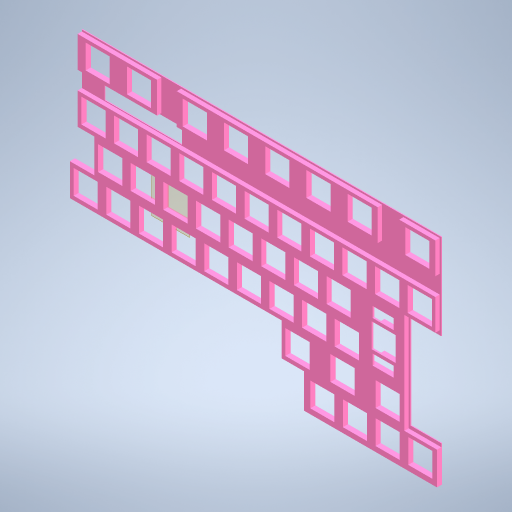
# Autodesk Inventor part: Upper Right Plate
Saved by Autodesk Inventor 2024 (Build 280153000, 153)
## iProperties
Created: 2024-06-29
Part Number: Upper Right Plate
Material: PET Plastic
Document SubType Name: Modeling
Designer: adam
Density: 1.541 g/cm^3
Appearance: Pink
Author: adam
Autodesk Inventor part; units mm, degrees
(part 1 of 2)
ref_plane "YZ Plane" through (0, 0, 0) normal (1, 0, 0) x (0, 1, 0)
ref_plane "XZ Plane" through (0, 0, 0) normal (0, 1, 0) x (-1, 0, 0)
ref_plane "XY Plane" through (0, 0, 0) normal (0, 0, 1) x (1, 0, 0)
sketch "Sketch1" plane through (0, 0, 0) normal (0, 0, 1) x (1, 0, 0)
  line L0 (43.325, -43.95) -> (49.375, -43.95) construction
  line L1 (49.375, -43.95) -> (49.375, -61) construction
  line L2 (49.375, -61) -> (43.325, -61) construction
  line L3 (43.325, -61) -> (43.325, -43.95) construction
  line L4 (117.95, -19.8) -> (117.95, -13.75) construction
  line L5 (117.95, -13.75) -> (135, -13.75) construction
  line L6 (135, -13.75) -> (135, -19.8) construction
  line L7 (135, -19.8) -> (117.95, -19.8) construction
  line L8 (26.325, -43.95) -> (32.375, -43.95) construction
  line L9 (32.375, -43.95) -> (32.375, -61) construction
  line L10 (32.375, -61) -> (26.325, -61) construction
  line L11 (26.325, -61) -> (26.325, -43.95) construction
  line L12 (-152.525, 13.425) -> (-146.475, 13.425) construction
  line L13 (-146.475, 13.425) -> (-146.475, -3.625) construction
  line L14 (-146.475, -3.625) -> (-152.525, -3.625) construction
  line L15 (-152.525, -3.625) -> (-152.525, 13.425) construction
  line L16 (-90.675, -43.95) -> (-84.625, -43.95) construction
  line L17 (-84.625, -43.95) -> (-84.625, -61) construction
  line L18 (-84.625, -61) -> (-90.675, -61) construction
  line L19 (-90.675, -61) -> (-90.675, -43.95) construction
  line L20 (39.375, -43.95) -> (39.375, -61) construction
  line L21 (39.375, -61) -> (33.325, -61) construction
  line L22 (33.325, -61) -> (33.325, -43.95) construction
  line L23 (33.325, -43.95) -> (39.375, -43.95) construction
  line L24 (117.95, 4.2) -> (117.95, 10.25) construction
  line L25 (117.95, 10.25) -> (135, 10.25) construction
  line L26 (135, 10.25) -> (135, 4.2) construction
  line L27 (135, 4.2) -> (117.95, 4.2) construction
  line L28 (-67.625, -43.95) -> (-67.625, -61) construction
  line L29 (-67.625, -61) -> (-73.675, -61) construction
  line L30 (-73.675, -61) -> (-73.675, -43.95) construction
  line L31 (-73.675, -43.95) -> (-67.625, -43.95) construction
  line L32 (-128.525, 13.425) -> (-122.475, 13.425) construction
  line L33 (-122.475, 13.425) -> (-122.475, -3.625) construction
  line L34 (-122.475, -3.625) -> (-128.525, -3.625) construction
  line L35 (-128.525, -3.625) -> (-128.525, 13.425) construction
  line L36 (-74.625, -43.95) -> (-74.625, -61) construction
  line L37 (-74.625, -61) -> (-80.675, -61) construction
  line L38 (-80.675, -61) -> (-80.675, -43.95) construction
  line L39 (-80.675, -43.95) -> (-74.625, -43.95) construction
  line L40 (-157.5, -62.5) -> (157.5, -62.5) construction
  line L41 (157.5, -62.5) -> (157.5, -41.5) construction
  line L42 (157.5, -41.5) -> (139.5, -41.5) construction
  line L43 (139.5, -41.5) -> (139.5, 12.5) construction
  line L44 (139.5, 12.5) -> (157.5, 12.5) construction
  line L45 (157.5, 12.5) -> (157.5, 62.5) construction
  line L46 (157.5, 62.5) -> (-157.5, 62.5) construction
  line L47 (-157.5, 62.5) -> (-157.5, -62.5) construction
  line L48 (-38.5, 42.5) -> (6.5, 42.5) construction
  line L49 (6.5, 42.5) -> (6.5, 33.5) construction
  line L50 (6.5, 33.5) -> (-38.5, 33.5) construction
  line L51 (-38.5, 33.5) -> (-38.5, 42.5) construction
  line L52 (154.775, -45.45) -> (154.775, -59.5) construction
  line L53 (154.775, -59.5) -> (140.725, -59.5) construction
  line L54 (140.725, -59.5) -> (140.725, -45.45) construction
  line L55 (140.725, -45.45) -> (154.775, -45.45) construction
  line L56 (135.775, -45.45) -> (135.775, -59.5) construction
  line L57 (135.775, -59.5) -> (121.725, -59.5) construction
  line L58 (121.725, -59.5) -> (121.725, -45.45) construction
  line L59 (121.725, -45.45) -> (135.775, -45.45) construction
  line L60 (116.775, -45.45) -> (116.775, -59.5) construction
  line L61 (116.775, -59.5) -> (102.725, -59.5) construction
  line L62 (102.725, -59.5) -> (102.725, -45.45) construction
  line L63 (102.725, -45.45) -> (116.775, -45.45) construction
  line L64 (97.775, -45.45) -> (97.775, -59.5) construction
  line L65 (97.775, -59.5) -> (83.725, -59.5) construction
  line L66 (83.725, -59.5) -> (83.725, -45.45) construction
  line L67 (83.725, -45.45) -> (97.775, -45.45) construction
  line L68 (75.775, -45.45) -> (75.775, -59.5) construction
  line L69 (75.775, -59.5) -> (61.725, -59.5) construction
  line L70 (61.725, -59.5) -> (61.725, -45.45) construction
  line L71 (61.725, -45.45) -> (75.775, -45.45) construction
  line L72 (-13.625, -45.45) -> (-13.625, -59.5) construction
  line L73 (-13.625, -59.5) -> (-27.675, -59.5) construction
  line L74 (-27.675, -59.5) -> (-27.675, -45.45) construction
  line L75 (-27.675, -45.45) -> (-13.625, -45.45) construction
  line L76 (-102.975, -45.45) -> (-102.975, -59.5) construction
  line L77 (-102.975, -59.5) -> (-117.025, -59.5) construction
  line L78 (-117.025, -59.5) -> (-117.025, -45.45) construction
  line L79 (-117.025, -45.45) -> (-102.975, -45.45) construction
  line L80 (-141.525, -45.45) -> (-127.475, -45.45) construction
  line L81 (-127.475, -45.45) -> (-127.475, -59.5) construction
  line L82 (-127.475, -59.5) -> (-141.525, -59.5) construction
  line L83 (-141.525, -59.5) -> (-141.525, -45.45) construction
  line L84 (121.725, -26.275) -> (135.775, -26.275) construction
  line L85 (135.775, -26.275) -> (135.775, -40.325) construction
  line L86 (135.775, -40.325) -> (121.725, -40.325) construction
  line L87 (121.725, -40.325) -> (121.725, -26.275) construction
  line L88 (95.475, -26.275) -> (109.525, -26.275) construction
  line L89 (109.525, -26.275) -> (109.525, -40.325) construction
  line L90 (109.525, -40.325) -> (95.475, -40.325) construction
  line L91 (95.475, -40.325) -> (95.475, -26.275) construction
  line L92 (69.225, -26.275) -> (83.275, -26.275) construction
  line L93 (83.275, -26.275) -> (83.275, -40.325) construction
  line L94 (83.275, -40.325) -> (69.225, -40.325) construction
  line L95 (69.225, -40.325) -> (69.225, -26.275) construction
  line L96 (50.225, -26.275) -> (64.275, -26.275) construction
  line L97 (64.275, -26.275) -> (64.275, -40.325) construction
  line L98 (64.275, -40.325) -> (50.225, -40.325) construction
  line L99 (50.225, -40.325) -> (50.225, -26.275) construction
  line L100 (31.225, -26.275) -> (45.275, -26.275) construction
  line L101 (45.275, -26.275) -> (45.275, -40.325) construction
  line L102 (45.275, -40.325) -> (31.225, -40.325) construction
  line L103 (31.225, -40.325) -> (31.225, -26.275) construction
  line L104 (12.225, -26.275) -> (26.275, -26.275) construction
  line L105 (26.275, -26.275) -> (26.275, -40.325) construction
  line L106 (26.275, -40.325) -> (12.225, -40.325) construction
  line L107 (12.225, -40.325) -> (12.225, -26.275) construction
  line L108 (-6.775, -26.275) -> (7.275, -26.275) construction
  line L109 (7.275, -26.275) -> (7.275, -40.325) construction
  line L110 (7.275, -40.325) -> (-6.775, -40.325) construction
  line L111 (-6.775, -40.325) -> (-6.775, -26.275) construction
  line L112 (-25.775, -26.275) -> (-11.725, -26.275) construction
  line L113 (-11.725, -26.275) -> (-11.725, -40.325) construction
  line L114 (-11.725, -40.325) -> (-25.775, -40.325) construction
  line L115 (-25.775, -40.325) -> (-25.775, -26.275) construction
  line L116 (-44.775, -26.275) -> (-30.725, -26.275) construction
  line L117 (-30.725, -26.275) -> (-30.725, -40.325) construction
  line L118 (-30.725, -40.325) -> (-44.775, -40.325) construction
  line L119 (-44.775, -40.325) -> (-44.775, -26.275) construction
  line L120 (-63.775, -26.275) -> (-49.725, -26.275) construction
  line L121 (-49.725, -26.275) -> (-49.725, -40.325) construction
  line L122 (-49.725, -40.325) -> (-63.775, -40.325) construction
  line L123 (-63.775, -40.325) -> (-63.775, -26.275) construction
  line L124 (-82.775, -26.275) -> (-68.725, -26.275) construction
  line L125 (-68.725, -26.275) -> (-68.725, -40.325) construction
  line L126 (-68.725, -40.325) -> (-82.775, -40.325) construction
  line L127 (-82.775, -40.325) -> (-82.775, -26.275) construction
  line L128 (-101.775, -26.275) -> (-87.725, -26.275) construction
  line L129 (-87.725, -26.275) -> (-87.725, -40.325) construction
  line L130 (-87.725, -40.325) -> (-101.775, -40.325) construction
  line L131 (-101.775, -40.325) -> (-101.775, -26.275) construction
  line L132 (-120.775, -26.275) -> (-106.725, -26.275) construction
  line L133 (-106.725, -26.275) -> (-106.725, -40.325) construction
  line L134 (-106.725, -40.325) -> (-120.775, -40.325) construction
  line L135 (-120.775, -40.325) -> (-120.775, -26.275) construction
  line L136 (-146.775, -26.275) -> (-132.725, -26.275) construction
  line L137 (-132.725, -26.275) -> (-132.725, -40.325) construction
  line L138 (-132.725, -40.325) -> (-146.775, -40.325) construction
  line L139 (-146.775, -40.325) -> (-146.775, -26.275) construction
  line L140 (97.975, -7.175) -> (112.025, -7.175) construction
  line L141 (112.025, -7.175) -> (112.025, -21.225) construction
  line L142 (112.025, -21.225) -> (97.975, -21.225) construction
  line L143 (97.975, -21.225) -> (97.975, -7.175) construction
  line L144 (78.975, -7.175) -> (93.025, -7.175) construction
  line L145 (93.025, -7.175) -> (93.025, -21.225) construction
  line L146 (93.025, -21.225) -> (78.975, -21.225) construction
  line L147 (78.975, -21.225) -> (78.975, -7.175) construction
  line L148 (59.975, -7.175) -> (74.025, -7.175) construction
  line L149 (74.025, -7.175) -> (74.025, -21.225) construction
  line L150 (74.025, -21.225) -> (59.975, -21.225) construction
  line L151 (59.975, -21.225) -> (59.975, -7.175) construction
  line L152 (40.975, -7.175) -> (55.025, -7.175) construction
  line L153 (55.025, -7.175) -> (55.025, -21.225) construction
  line L154 (55.025, -21.225) -> (40.975, -21.225) construction
  line L155 (40.975, -21.225) -> (40.975, -7.175) construction
  line L156 (21.975, -7.175) -> (36.025, -7.175) construction
  line L157 (36.025, -7.175) -> (36.025, -21.225) construction
  line L158 (36.025, -21.225) -> (21.975, -21.225) construction
  line L159 (21.975, -21.225) -> (21.975, -7.175) construction
  line L160 (2.975, -7.175) -> (17.025, -7.175) construction
  line L161 (17.025, -7.175) -> (17.025, -21.225) construction
  line L162 (17.025, -21.225) -> (2.975, -21.225) construction
  line L163 (2.975, -21.225) -> (2.975, -7.175) construction
  line L164 (-16.025, -7.175) -> (-1.975, -7.175) construction
  line L165 (-1.975, -7.175) -> (-1.975, -21.225) construction
  line L166 (-1.975, -21.225) -> (-16.025, -21.225) construction
  line L167 (-16.025, -21.225) -> (-16.025, -7.175) construction
  line L168 (-35.025, -7.175) -> (-20.975, -7.175) construction
  line L169 (-20.975, -7.175) -> (-20.975, -21.225) construction
  line L170 (-20.975, -21.225) -> (-35.025, -21.225) construction
  line L171 (-35.025, -21.225) -> (-35.025, -7.175) construction
  line L172 (-54.025, -7.175) -> (-39.975, -7.175) construction
  line L173 (-39.975, -7.175) -> (-39.975, -21.225) construction
  line L174 (-39.975, -21.225) -> (-54.025, -21.225) construction
  line L175 (-54.025, -21.225) -> (-54.025, -7.175) construction
  line L176 (-73.025, -7.175) -> (-58.975, -7.175) construction
  line L177 (-58.975, -7.175) -> (-58.975, -21.225) construction
  line L178 (-58.975, -21.225) -> (-73.025, -21.225) construction
  line L179 (-73.025, -21.225) -> (-73.025, -7.175) construction
  line L180 (-92.025, -7.175) -> (-77.975, -7.175) construction
  line L181 (-77.975, -7.175) -> (-77.975, -21.225) construction
  line L182 (-77.975, -21.225) -> (-92.025, -21.225) construction
  line L183 (-92.025, -21.225) -> (-92.025, -7.175) construction
  line L184 (-111.025, -7.175) -> (-96.975, -7.175) construction
  line L185 (-96.975, -7.175) -> (-96.975, -21.225) construction
  line L186 (-96.975, -21.225) -> (-111.025, -21.225) construction
  line L187 (-111.025, -21.225) -> (-111.025, -7.175) construction
  line L188 (-130.025, -7.175) -> (-115.975, -7.175) construction
  line L189 (-115.975, -7.175) -> (-115.975, -21.225) construction
  line L190 (-115.975, -21.225) -> (-130.025, -21.225) construction
  line L191 (-130.025, -21.225) -> (-130.025, -7.175) construction
  line L192 (-151.525, -7.175) -> (-137.475, -7.175) construction
  line L193 (-137.475, -7.175) -> (-137.475, -21.225) construction
  line L194 (-137.475, -21.225) -> (-151.525, -21.225) construction
  line L195 (-151.525, -21.225) -> (-151.525, -7.175) construction
  line L196 (119.45, 2.25) -> (133.5, 2.25) construction
  line L197 (133.5, 2.25) -> (133.5, -11.8) construction
  line L198 (133.5, -11.8) -> (119.45, -11.8) construction
  line L199 (119.45, -11.8) -> (119.45, 2.25) construction
  line L200 (107.275, 11.925) -> (107.275, -2.125) construction
  line L201 (107.275, -2.125) -> (93.225, -2.125) construction
  line L202 (93.225, -2.125) -> (93.225, 11.925) construction
  line L203 (93.225, 11.925) -> (107.275, 11.925) construction
  line L204 (88.275, 11.925) -> (88.275, -2.125) construction
  line L205 (88.275, -2.125) -> (74.225, -2.125) construction
  line L206 (74.225, -2.125) -> (74.225, 11.925) construction
  line L207 (74.225, 11.925) -> (88.275, 11.925) construction
  line L208 (69.275, 11.925) -> (69.275, -2.125) construction
  line L209 (69.275, -2.125) -> (55.225, -2.125) construction
  line L210 (55.225, -2.125) -> (55.225, 11.925) construction
  line L211 (55.225, 11.925) -> (69.275, 11.925) construction
  line L212 (50.275, 11.925) -> (50.275, -2.125) construction
  line L213 (50.275, -2.125) -> (36.225, -2.125) construction
  line L214 (36.225, -2.125) -> (36.225, 11.925) construction
  line L215 (36.225, 11.925) -> (50.275, 11.925) construction
  line L216 (31.275, 11.925) -> (31.275, -2.125) construction
  line L217 (31.275, -2.125) -> (17.225, -2.125) construction
  line L218 (17.225, -2.125) -> (17.225, 11.925) construction
  line L219 (17.225, 11.925) -> (31.275, 11.925) construction
  line L220 (12.275, 11.925) -> (12.275, -2.125) construction
  line L221 (12.275, -2.125) -> (-1.775, -2.125) construction
  line L222 (-1.775, -2.125) -> (-1.775, 11.925) construction
  line L223 (-1.775, 11.925) -> (12.275, 11.925) construction
  line L224 (-6.725, 11.925) -> (-6.725, -2.125) construction
  line L225 (-6.725, -2.125) -> (-20.775, -2.125) construction
  line L226 (-20.775, -2.125) -> (-20.775, 11.925) construction
  line L227 (-20.775, 11.925) -> (-6.725, 11.925) construction
  line L228 (-25.725, 11.925) -> (-25.725, -2.125) construction
  line L229 (-25.725, -2.125) -> (-39.775, -2.125) construction
  line L230 (-39.775, -2.125) -> (-39.775, 11.925) construction
  line L231 (-39.775, 11.925) -> (-25.725, 11.925) construction
  line L232 (-44.725, 11.925) -> (-44.725, -2.125) construction
  line L233 (-44.725, -2.125) -> (-58.775, -2.125) construction
  line L234 (-58.775, -2.125) -> (-58.775, 11.925) construction
  line L235 (-58.775, 11.925) -> (-44.725, 11.925) construction
  line L236 (-63.725, 11.925) -> (-63.725, -2.125) construction
  line L237 (-63.725, -2.125) -> (-77.775, -2.125) construction
  line L238 (-77.775, -2.125) -> (-77.775, 11.925) construction
  line L239 (-77.775, 11.925) -> (-63.725, 11.925) construction
  line L240 (-82.725, 11.925) -> (-82.725, -2.125) construction
  line L241 (-82.725, -2.125) -> (-96.775, -2.125) construction
  line L242 (-96.775, -2.125) -> (-96.775, 11.925) construction
  line L243 (-96.775, 11.925) -> (-82.725, 11.925) construction
  line L244 (-101.725, 11.925) -> (-101.725, -2.125) construction
  line L245 (-101.725, -2.125) -> (-115.775, -2.125) construction
  line L246 (-115.775, -2.125) -> (-115.775, 11.925) construction
  line L247 (-115.775, 11.925) -> (-101.725, 11.925) construction
  line L248 (-144.525, 11.925) -> (-130.475, 11.925) construction
  line L249 (-130.475, 11.925) -> (-130.475, -2.125) construction
  line L250 (-130.475, -2.125) -> (-144.525, -2.125) construction
  line L251 (-144.525, -2.125) -> (-144.525, 11.925) construction
  line L252 (154.525, 16.975) -> (140.475, 16.975) construction
  line L253 (140.475, 16.975) -> (140.475, 31.025) construction
  line L254 (140.475, 31.025) -> (154.525, 31.025) construction
  line L255 (154.525, 31.025) -> (154.525, 16.975) construction
  line L256 (135.525, 16.975) -> (121.475, 16.975) construction
  line L257 (121.475, 16.975) -> (121.475, 31.025) construction
  line L258 (121.475, 31.025) -> (135.525, 31.025) construction
  line L259 (135.525, 31.025) -> (135.525, 16.975) construction
  line L260 (116.525, 16.975) -> (102.475, 16.975) construction
  line L261 (102.475, 16.975) -> (102.475, 31.025) construction
  line L262 (102.475, 31.025) -> (116.525, 31.025) construction
  line L263 (116.525, 31.025) -> (116.525, 16.975) construction
  line L264 (97.525, 16.975) -> (83.475, 16.975) construction
  line L265 (83.475, 16.975) -> (83.475, 31.025) construction
  line L266 (83.475, 31.025) -> (97.525, 31.025) construction
  line L267 (97.525, 31.025) -> (97.525, 16.975) construction
  line L268 (78.525, 16.975) -> (64.475, 16.975) construction
  line L269 (64.475, 16.975) -> (64.475, 31.025) construction
  line L270 (64.475, 31.025) -> (78.525, 31.025) construction
  line L271 (78.525, 31.025) -> (78.525, 16.975) construction
  line L272 (59.525, 16.975) -> (45.475, 16.975) construction
  line L273 (45.475, 16.975) -> (45.475, 31.025) construction
  line L274 (45.475, 31.025) -> (59.525, 31.025) construction
  line L275 (59.525, 31.025) -> (59.525, 16.975) construction
  line L276 (40.525, 16.975) -> (26.475, 16.975) construction
  line L277 (26.475, 16.975) -> (26.475, 31.025) construction
  line L278 (26.475, 31.025) -> (40.525, 31.025) construction
  line L279 (40.525, 31.025) -> (40.525, 16.975) construction
  line L280 (21.525, 16.975) -> (7.475, 16.975) construction
  line L281 (7.475, 16.975) -> (7.475, 31.025) construction
  line L282 (7.475, 31.025) -> (21.525, 31.025) construction
  line L283 (21.525, 31.025) -> (21.525, 16.975) construction
  line L284 (2.525, 16.975) -> (-11.525, 16.975) construction
  line L285 (-11.525, 16.975) -> (-11.525, 31.025) construction
  line L286 (-11.525, 31.025) -> (2.525, 31.025) construction
  line L287 (2.525, 31.025) -> (2.525, 16.975) construction
  line L288 (-16.475, 16.975) -> (-30.525, 16.975) construction
  line L289 (-30.525, 16.975) -> (-30.525, 31.025) construction
  line L290 (-30.525, 31.025) -> (-16.475, 31.025) construction
  line L291 (-16.475, 31.025) -> (-16.475, 16.975) construction
  line L292 (-35.475, 16.975) -> (-49.525, 16.975) construction
  line L293 (-49.525, 16.975) -> (-49.525, 31.025) construction
  line L294 (-49.525, 31.025) -> (-35.475, 31.025) construction
  line L295 (-35.475, 31.025) -> (-35.475, 16.975) construction
  line L296 (-54.475, 16.975) -> (-68.525, 16.975) construction
  line L297 (-68.525, 16.975) -> (-68.525, 31.025) construction
  line L298 (-68.525, 31.025) -> (-54.475, 31.025) construction
  line L299 (-54.475, 31.025) -> (-54.475, 16.975) construction
  line L300 (-73.475, 16.975) -> (-87.525, 16.975) construction
  line L301 (-87.525, 16.975) -> (-87.525, 31.025) construction
  line L302 (-87.525, 31.025) -> (-73.475, 31.025) construction
  line L303 (-73.475, 31.025) -> (-73.475, 16.975) construction
  line L304 (-92.475, 16.975) -> (-106.525, 16.975) construction
  line L305 (-106.525, 16.975) -> (-106.525, 31.025) construction
  line L306 (-106.525, 31.025) -> (-92.475, 31.025) construction
  line L307 (-92.475, 31.025) -> (-92.475, 16.975) construction
  line L308 (-111.475, 16.975) -> (-125.525, 16.975) construction
  line L309 (-125.525, 16.975) -> (-125.525, 31.025) construction
  line L310 (-125.525, 31.025) -> (-111.475, 31.025) construction
  line L311 (-111.475, 31.025) -> (-111.475, 16.975) construction
  line L312 (-149.525, 31.025) -> (-135.475, 31.025) construction
  line L313 (-135.475, 31.025) -> (-135.475, 16.975) construction
  line L314 (-135.475, 16.975) -> (-149.525, 16.975) construction
  line L315 (-149.525, 16.975) -> (-149.525, 31.025) construction
  line L316 (138.975, 59.525) -> (153.025, 59.525) construction
  line L317 (153.025, 59.525) -> (153.025, 45.475) construction
  line L318 (153.025, 45.475) -> (138.975, 45.475) construction
  line L319 (138.975, 45.475) -> (138.975, 59.525) construction
  line L320 (105.475, 59.525) -> (119.525, 59.525) construction
  line L321 (119.525, 59.525) -> (119.525, 45.475) construction
  line L322 (119.525, 45.475) -> (105.475, 45.475) construction
  line L323 (105.475, 45.475) -> (105.475, 59.525) construction
  line L324 (81.475, 59.525) -> (95.525, 59.525) construction
  line L325 (95.525, 59.525) -> (95.525, 45.475) construction
  line L326 (95.525, 45.475) -> (81.475, 45.475) construction
  line L327 (81.475, 45.475) -> (81.475, 59.525) construction
  line L328 (57.475, 59.525) -> (71.525, 59.525) construction
  line L329 (71.525, 59.525) -> (71.525, 45.475) construction
  line L330 (71.525, 45.475) -> (57.475, 45.475) construction
  line L331 (57.475, 45.475) -> (57.475, 59.525) construction
  line L332 (33.475, 59.525) -> (47.525, 59.525) construction
  line L333 (47.525, 59.525) -> (47.525, 45.475) construction
  line L334 (47.525, 45.475) -> (33.475, 45.475) construction
  line L335 (33.475, 45.475) -> (33.475, 59.525) construction
  line L336 (9.475, 59.525) -> (23.525, 59.525) construction
  line L337 (23.525, 59.525) -> (23.525, 45.475) construction
  line L338 (23.525, 45.475) -> (9.475, 45.475) construction
  line L339 (9.475, 45.475) -> (9.475, 59.525) construction
  line L340 (-23.025, 59.525) -> (-8.975, 59.525) construction
  line L341 (-8.975, 59.525) -> (-8.975, 45.475) construction
  line L342 (-8.975, 45.475) -> (-23.025, 45.475) construction
  line L343 (-23.025, 45.475) -> (-23.025, 59.525) construction
  line L344 (-47.025, 59.525) -> (-32.975, 59.525) construction
  line L345 (-32.975, 59.525) -> (-32.975, 45.475) construction
  line L346 (-32.975, 45.475) -> (-47.025, 45.475) construction
  line L347 (-47.025, 45.475) -> (-47.025, 59.525) construction
  line L348 (-71.025, 59.525) -> (-56.975, 59.525) construction
  line L349 (-56.975, 59.525) -> (-56.975, 45.475) construction
  line L350 (-56.975, 45.475) -> (-71.025, 45.475) construction
  line L351 (-71.025, 45.475) -> (-71.025, 59.525) construction
  line L352 (-95.025, 59.525) -> (-80.975, 59.525) construction
  line L353 (-80.975, 59.525) -> (-80.975, 45.475) construction
  line L354 (-80.975, 45.475) -> (-95.025, 45.475) construction
  line L355 (-95.025, 45.475) -> (-95.025, 59.525) construction
  line L356 (-119.025, 59.525) -> (-104.975, 59.525) construction
  line L357 (-104.975, 59.525) -> (-104.975, 45.475) construction
  line L358 (-104.975, 45.475) -> (-119.025, 45.475) construction
  line L359 (-119.025, 45.475) -> (-119.025, 59.525) construction
  line L360 (-152.025, 59.525) -> (-137.975, 59.525) construction
  line L361 (-137.975, 59.525) -> (-137.975, 45.475) construction
  line L362 (-137.975, 45.475) -> (-152.025, 45.475) construction
  line L363 (-152.025, 45.475) -> (-152.025, 59.525) construction
  line L364 (79.5, -62.5) -> (79.5, -43.1375) construction
  line L365 (79.5, -43.1375) -> (66.5, -43.1375) construction
  line L366 (66.5, -43.1375) -> (66.5, -24) construction
  line L367 (66.5, -24) -> (-104, -24) construction
  line L368 (-104, -24) -> (-104, -43.1375) construction
  line L369 (-104, -43.1375) -> (-122, -43.1375) construction
  line L370 (-122, -43.1375) -> (-122, -62.5) construction
  line L371 (-122, -62.5) -> (79.5, -62.5) construction
  line L372 (43.325, -58.35) -> (43.325, -45.95) construction
  line L373 (43.325, -45.95) -> (49.375, -45.95) construction
  line L374 (49.375, -45.95) -> (49.375, -58.35) construction
  line L375 (49.375, -58.35) -> (43.325, -58.35) construction
  line L376 (-90.675, -58.35) -> (-90.675, -45.95) construction
  line L377 (-90.675, -45.95) -> (-84.625, -45.95) construction
  line L378 (-84.625, -45.95) -> (-84.625, -58.35) construction
  line L379 (-84.625, -58.35) -> (-90.675, -58.35) construction
  line L380 (61.725, -45.45) -> (75.775, -45.45) construction
  line L381 (75.775, -45.45) -> (75.775, -59.5) construction
  line L382 (75.775, -59.5) -> (61.725, -59.5) construction
  line L383 (61.725, -59.5) -> (61.725, -45.45) construction
  line L384 (50.225, -26.275) -> (64.275, -26.275) construction
  line L385 (64.275, -26.275) -> (64.275, -40.325) construction
  line L386 (64.275, -40.325) -> (50.225, -40.325) construction
  line L387 (50.225, -40.325) -> (50.225, -26.275) construction
  line L388 (31.225, -26.275) -> (45.275, -26.275) construction
  line L389 (45.275, -26.275) -> (45.275, -40.325) construction
  line L390 (45.275, -40.325) -> (31.225, -40.325) construction
  line L391 (31.225, -40.325) -> (31.225, -26.275) construction
  line L392 (12.225, -40.325) -> (12.225, -26.275) construction
  line L393 (12.225, -26.275) -> (26.275, -26.275) construction
  line L394 (26.275, -26.275) -> (26.275, -40.325) construction
  line L395 (26.275, -40.325) -> (12.225, -40.325) construction
  line L396 (-6.775, -40.325) -> (-6.775, -26.275) construction
  line L397 (-6.775, -26.275) -> (7.275, -26.275) construction
  line L398 (7.275, -26.275) -> (7.275, -40.325) construction
  line L399 (7.275, -40.325) -> (-6.775, -40.325) construction
  line L400 (-27.675, -45.45) -> (-13.625, -45.45) construction
  line L401 (-13.625, -45.45) -> (-13.625, -59.5) construction
  line L402 (-13.625, -59.5) -> (-27.675, -59.5) construction
  line L403 (-27.675, -59.5) -> (-27.675, -45.45) construction
  line L404 (-25.775, -26.275) -> (-11.725, -26.275) construction
  line L405 (-11.725, -26.275) -> (-11.725, -40.325) construction
  line L406 (-11.725, -40.325) -> (-25.775, -40.325) construction
  line L407 (-25.775, -40.325) -> (-25.775, -26.275) construction
  line L408 (-44.775, -40.325) -> (-44.775, -26.275) construction
  line L409 (-44.775, -26.275) -> (-30.725, -26.275) construction
  line L410 (-30.725, -26.275) -> (-30.725, -40.325) construction
  line L411 (-30.725, -40.325) -> (-44.775, -40.325) construction
  line L412 (-49.725, -40.325) -> (-63.775, -40.325) construction
  line L413 (-63.775, -40.325) -> (-63.775, -26.275) construction
  line L414 (-63.775, -26.275) -> (-49.725, -26.275) construction
  line L415 (-49.725, -26.275) -> (-49.725, -40.325) construction
  line L416 (-82.775, -40.325) -> (-82.775, -26.275) construction
  line L417 (-82.775, -26.275) -> (-68.725, -26.275) construction
  line L418 (-68.725, -26.275) -> (-68.725, -40.325) construction
  line L419 (-68.725, -40.325) -> (-82.775, -40.325) construction
  line L420 (-87.725, -40.325) -> (-101.775, -40.325) construction
  line L421 (-101.775, -40.325) -> (-101.775, -26.275) construction
  line L422 (-101.775, -26.275) -> (-87.725, -26.275) construction
  line L423 (-87.725, -26.275) -> (-87.725, -40.325) construction
  line L424 (-102.975, -45.45) -> (-102.975, -59.5) construction
  line L425 (-102.975, -59.5) -> (-117.025, -59.5) construction
  line L426 (-117.025, -59.5) -> (-117.025, -45.45) construction
  line L427 (-117.025, -45.45) -> (-102.975, -45.45) construction
  line L428 (-52, 62.5) -> (-52, 14.45) construction
  line L429 (-52, 14.45) -> (-42.25, 14.45) construction
  line L430 (-42.25, 14.45) -> (-42.25, -4.65) construction
  line L431 (-42.25, -4.65) -> (-56.5, -4.65) construction
  line L432 (-56.5, -4.65) -> (-56.5, -24) construction
  line L433 (-54.475, 31.025) -> (-52, 31.025) construction
  line L434 (-52, 31.025) -> (-49.525, 31.025) construction
  line L435 (-49.525, 16.975) -> (-49.525, 14.45) construction
  line L436 (-49.525, 14.45) -> (-49.525, 11.925) construction
  line L437 (-44.725, 11.925) -> (-42.25, 11.925) construction
  line L438 (-42.25, 11.925) -> (-39.775, 11.925) construction
  line L439 (-44.725, -2.125) -> (-44.725, -4.65) construction
  line L440 (-44.725, -4.65) -> (-44.725, -7.175) construction
  line L441 (-58.975, -7.175) -> (-56.5, -7.175) construction
  line L442 (-56.5, -7.175) -> (-54.025, -7.175) construction
  line L443 (-51.75, 62.5) -> (-51.75, 14.7)
  line L444 (-51.75, 14.7) -> (-42, 14.7)
  line L445 (-42, 14.7) -> (-42, -4.9)
  line L446 (-42, -4.9) -> (-56.25, -4.9)
  line L447 (-56.25, -4.9) -> (-56.25, -23.5)
  line L448 (-56.25, -23.5) -> (67, -23.5)
  line L449 (67, -23.5) -> (67, -42.6375)
  line L450 (67, -42.6375) -> (80, -42.6375)
  line L451 (80, -42.6375) -> (80, -62.5)
  line L452 (80, -62.5) -> (157.5, -62.5)
  line L453 (157.5, -62.5) -> (157.5, -41.5)
  line L454 (157.5, 12.5) -> (157.5, 62.5)
  line L455 (157.5, 62.5) -> (-51.75, 62.5)
  line L456 (157.5, 12.5) -> (139.5, 12.5)
  line L457 (139.5, 12.5) -> (139.5, -41.5)
  line L458 (139.5, -41.5) -> (157.5, -41.5)
  line L459 (-38.5, 42.5) -> (6.5, 42.5) projected
  line L460 (-38.5, 33.5) -> (-38.5, 42.5) projected
  line L461 (6.5, 33.5) -> (-38.5, 33.5) projected
  line L462 (6.5, 42.5) -> (6.5, 33.5) projected
  line L463 (23.525, 45.475) -> (9.475, 45.475) projected
  line L464 (23.525, 59.525) -> (23.525, 45.475) projected
  line L465 (9.475, 59.525) -> (23.525, 59.525) projected
  line L466 (9.475, 45.475) -> (9.475, 59.525) projected
  line L467 (-23.025, 59.525) -> (-8.975, 59.525) projected
  line L468 (-8.975, 59.525) -> (-8.975, 45.475) projected
  line L469 (-23.025, 45.475) -> (-23.025, 59.525) projected
  line L470 (-8.975, 45.475) -> (-23.025, 45.475) projected
  line L471 (-32.975, 59.525) -> (-32.975, 45.475) projected
  line L472 (-47.025, 59.525) -> (-32.975, 59.525) projected
  line L473 (-47.025, 45.475) -> (-47.025, 59.525) projected
  line L474 (-32.975, 45.475) -> (-47.025, 45.475) projected
  line L475 (-49.525, 31.025) -> (-35.475, 31.025) projected
  line L476 (-35.475, 31.025) -> (-35.475, 16.975) projected
  line L477 (-49.525, 16.975) -> (-49.525, 31.025) projected
  line L478 (-35.475, 16.975) -> (-49.525, 16.975) projected
  line L479 (-16.475, 16.975) -> (-30.525, 16.975) projected
  line L480 (-30.525, 16.975) -> (-30.525, 31.025) projected
  line L481 (-30.525, 31.025) -> (-16.475, 31.025) projected
  line L482 (-16.475, 31.025) -> (-16.475, 16.975) projected
  line L483 (-11.525, 16.975) -> (-11.525, 31.025) projected
  line L484 (-11.525, 31.025) -> (2.525, 31.025) projected
  line L485 (2.525, 31.025) -> (2.525, 16.975) projected
  line L486 (2.525, 16.975) -> (-11.525, 16.975) projected
  line L487 (21.525, 16.975) -> (7.475, 16.975) projected
  line L488 (7.475, 31.025) -> (21.525, 31.025) projected
  line L489 (21.525, 31.025) -> (21.525, 16.975) projected
  line L490 (33.475, 59.525) -> (47.525, 59.525) projected
  line L491 (47.525, 59.525) -> (47.525, 45.475) projected
  line L492 (47.525, 45.475) -> (33.475, 45.475) projected
  line L493 (57.475, 45.475) -> (57.475, 59.525) projected
  line L494 (57.475, 59.525) -> (71.525, 59.525) projected
  line L495 (71.525, 59.525) -> (71.525, 45.475) projected
  line L496 (71.525, 45.475) -> (57.475, 45.475) projected
  line L497 (81.475, 59.525) -> (95.525, 59.525) projected
  line L498 (95.525, 59.525) -> (95.525, 45.475) projected
  line L499 (81.475, 45.475) -> (81.475, 59.525) projected
  line L500 (95.525, 45.475) -> (81.475, 45.475) projected
  line L501 (105.475, 45.475) -> (105.475, 59.525) projected
  line L502 (105.475, 59.525) -> (119.525, 59.525) projected
  line L503 (119.525, 59.525) -> (119.525, 45.475) projected
  line L504 (119.525, 45.475) -> (105.475, 45.475) projected
  line L505 (138.975, 45.475) -> (138.975, 59.525) projected
  line L506 (138.975, 59.525) -> (153.025, 59.525) projected
  line L507 (153.025, 59.525) -> (153.025, 45.475) projected
  line L508 (153.025, 45.475) -> (138.975, 45.475) projected
  line L509 (26.475, 31.025) -> (40.525, 31.025) projected
  line L510 (40.525, 31.025) -> (40.525, 16.975) projected
  line L511 (40.525, 16.975) -> (26.475, 16.975) projected
  line L512 (26.475, 16.975) -> (26.475, 31.025) projected
  line L513 (45.475, 31.025) -> (59.525, 31.025) projected
  line L514 (45.475, 16.975) -> (45.475, 31.025) projected
  line L515 (59.525, 31.025) -> (59.525, 16.975) projected
  line L516 (59.525, 16.975) -> (45.475, 16.975) projected
  line L517 (64.475, 31.025) -> (78.525, 31.025) projected
  line L518 (78.525, 31.025) -> (78.525, 16.975) projected
  line L519 (64.475, 16.975) -> (64.475, 31.025) projected
  line L520 (78.525, 16.975) -> (64.475, 16.975) projected
  line L521 (83.475, 16.975) -> (83.475, 31.025) projected
  line L522 (97.525, 16.975) -> (83.475, 16.975) projected
  line L523 (97.525, 31.025) -> (97.525, 16.975) projected
  line L524 (83.475, 31.025) -> (97.525, 31.025) projected
  line L525 (102.475, 31.025) -> (116.525, 31.025) projected
  line L526 (116.525, 31.025) -> (116.525, 16.975) projected
  line L527 (102.475, 16.975) -> (102.475, 31.025) projected
  line L528 (116.525, 16.975) -> (102.475, 16.975) projected
  line L529 (121.475, 31.025) -> (135.525, 31.025) projected
  line L530 (135.525, 31.025) -> (135.525, 16.975) projected
  line L531 (121.475, 16.975) -> (121.475, 31.025) projected
  line L532 (135.525, 16.975) -> (121.475, 16.975) projected
  line L533 (140.475, 31.025) -> (154.525, 31.025) projected
  line L534 (154.525, 31.025) -> (154.525, 16.975) projected
  line L535 (154.525, 16.975) -> (140.475, 16.975) projected
  line L536 (140.475, 16.975) -> (140.475, 31.025) projected
  line L537 (17.225, 11.925) -> (31.275, 11.925) projected
  line L538 (31.275, 11.925) -> (31.275, -2.125) projected
  line L539 (17.225, -2.125) -> (17.225, 11.925) projected
  line L540 (31.275, -2.125) -> (17.225, -2.125) projected
  line L541 (36.225, 11.925) -> (50.275, 11.925) projected
  line L542 (50.275, 11.925) -> (50.275, -2.125) projected
  line L543 (36.225, -2.125) -> (36.225, 11.925) projected
  line L544 (50.275, -2.125) -> (36.225, -2.125) projected
  line L545 (55.225, 11.925) -> (69.275, 11.925) projected
  line L546 (69.275, 11.925) -> (69.275, -2.125) projected
  line L547 (55.225, -2.125) -> (55.225, 11.925) projected
  line L548 (69.275, -2.125) -> (55.225, -2.125) projected
  line L549 (74.225, 11.925) -> (88.275, 11.925) projected
  line L550 (88.275, 11.925) -> (88.275, -2.125) projected
  line L551 (74.225, -2.125) -> (74.225, 11.925) projected
  line L552 (88.275, -2.125) -> (74.225, -2.125) projected
  line L553 (93.225, -2.125) -> (93.225, 11.925) projected
  line L554 (93.225, 11.925) -> (107.275, 11.925) projected
  line L555 (107.275, 11.925) -> (107.275, -2.125) projected
  line L556 (107.275, -2.125) -> (93.225, -2.125) projected
  line L557 (21.975, -7.175) -> (36.025, -7.175) projected
  line L558 (36.025, -7.175) -> (36.025, -21.225) projected
  line L559 (21.975, -21.225) -> (21.975, -7.175) projected
  line L560 (36.025, -21.225) -> (21.975, -21.225) projected
  line L561 (40.975, -7.175) -> (55.025, -7.175) projected
  line L562 (55.025, -7.175) -> (55.025, -21.225) projected
  line L563 (40.975, -21.225) -> (40.975, -7.175) projected
  line L564 (55.025, -21.225) -> (40.975, -21.225) projected
  line L565 (59.975, -21.225) -> (59.975, -7.175) projected
  line L566 (74.025, -21.225) -> (59.975, -21.225) projected
  line L567 (74.025, -7.175) -> (74.025, -21.225) projected
  line L568 (59.975, -7.175) -> (74.025, -7.175) projected
  line L569 (78.975, -7.175) -> (93.025, -7.175) projected
  line L570 (93.025, -7.175) -> (93.025, -21.225) projected
  line L571 (93.025, -21.225) -> (78.975, -21.225) projected
  line L572 (78.975, -21.225) -> (78.975, -7.175) projected
  line L573 (97.975, -7.175) -> (112.025, -7.175) projected
  line L574 (112.025, -7.175) -> (112.025, -21.225) projected
  line L575 (112.025, -21.225) -> (97.975, -21.225) projected
  line L576 (97.975, -21.225) -> (97.975, -7.175) projected
  line L577 (69.225, -26.275) -> (83.275, -26.275) projected
  line L578 (83.275, -26.275) -> (83.275, -40.325) projected
  line L579 (83.275, -40.325) -> (69.225, -40.325) projected
  line L580 (69.225, -40.325) -> (69.225, -26.275) projected
  line L581 (95.475, -40.325) -> (95.475, -26.275) projected
  line L582 (95.475, -26.275) -> (109.525, -26.275) projected
  line L583 (109.525, -26.275) -> (109.525, -40.325) projected
  line L584 (109.525, -40.325) -> (95.475, -40.325) projected
  line L585 (121.725, -40.325) -> (121.725, -26.275) projected
  line L586 (121.725, -26.275) -> (135.775, -26.275) projected
  line L587 (135.775, -26.275) -> (135.775, -40.325) projected
  line L588 (135.775, -40.325) -> (121.725, -40.325) projected
  line L589 (140.725, -45.45) -> (154.775, -45.45) projected
  line L590 (154.775, -45.45) -> (154.775, -59.5) projected
  line L591 (154.775, -59.5) -> (140.725, -59.5) projected
  line L592 (140.725, -59.5) -> (140.725, -45.45) projected
  line L593 (135.775, -45.45) -> (135.775, -59.5) projected
  line L594 (135.775, -59.5) -> (121.725, -59.5) projected
  line L595 (121.725, -59.5) -> (121.725, -45.45) projected
  line L596 (121.725, -45.45) -> (135.775, -45.45) projected
  line L597 (102.725, -45.45) -> (116.775, -45.45) projected
  line L598 (116.775, -45.45) -> (116.775, -59.5) projected
  line L599 (116.775, -59.5) -> (102.725, -59.5) projected
  line L600 (102.725, -59.5) -> (102.725, -45.45) projected
  line L601 (83.725, -45.45) -> (97.775, -45.45) projected
  line L602 (97.775, -45.45) -> (97.775, -59.5) projected
  line L603 (83.725, -59.5) -> (83.725, -45.45) projected
  line L604 (97.775, -59.5) -> (83.725, -59.5) projected
  line L605 (119.45, 2.25) -> (133.5, 2.25) projected
  line L606 (133.5, 2.25) -> (133.5, -11.8) projected
  line L607 (133.5, -11.8) -> (119.45, -11.8) projected
  line L608 (119.45, -11.8) -> (119.45, 2.25) projected
  line L609 (2.975, -7.175) -> (17.025, -7.175) projected
  line L610 (17.025, -7.175) -> (17.025, -21.225) projected
  line L611 (17.025, -21.225) -> (2.975, -21.225) projected
  line L612 (2.975, -21.225) -> (2.975, -7.175) projected
  line L613 (-1.975, -7.175) -> (-1.975, -21.225) projected
  line L614 (-16.025, -21.225) -> (-16.025, -7.175) projected
  line L615 (-16.025, -7.175) -> (-1.975, -7.175) projected
  line L616 (-1.975, -21.225) -> (-16.025, -21.225) projected
  line L617 (-1.775, 11.925) -> (12.275, 11.925) projected
  line L618 (12.275, -2.125) -> (-1.775, -2.125) projected
  line L619 (12.275, 11.925) -> (12.275, -2.125) projected
  line L620 (-1.775, -2.125) -> (-1.775, 11.925) projected
  line L621 (-20.775, 11.925) -> (-6.725, 11.925) projected
  line L622 (-6.725, 11.925) -> (-6.725, -2.125) projected
  line L623 (-20.775, -2.125) -> (-20.775, 11.925) projected
  line L624 (-6.725, -2.125) -> (-20.775, -2.125) projected
  line L625 (-25.725, 11.925) -> (-25.725, -2.125) projected
  line L626 (-39.775, -2.125) -> (-39.775, 11.925) projected
  line L627 (-25.725, -2.125) -> (-39.775, -2.125) projected
  line L628 (-54.025, -7.175) -> (-39.975, -7.175) projected
  line L629 (-39.975, -7.175) -> (-39.975, -21.225) projected
  line L630 (-54.025, -21.225) -> (-54.025, -7.175) projected
  line L631 (-39.975, -21.225) -> (-54.025, -21.225) projected
  line L632 (-35.025, -21.225) -> (-35.025, -7.175) projected
  line L633 (-35.025, -7.175) -> (-20.975, -7.175) projected
  line L634 (-20.975, -7.175) -> (-20.975, -21.225) projected
  line L635 (-20.975, -21.225) -> (-35.025, -21.225) projected
  line L636 (119.95, 10.25) -> (132.35, 10.25)
  line L637 (132.35, 10.25) -> (132.35, 4.2)
  line L638 (132.35, 4.2) -> (119.95, 4.2)
  line L639 (119.95, 4.2) -> (119.95, 10.25)
  line L640 (119.95, -13.75) -> (132.35, -13.75)
  line L641 (132.35, -13.75) -> (132.35, -19.8)
  line L642 (132.35, -19.8) -> (119.95, -19.8)
  line L643 (119.95, -19.8) -> (119.95, -13.75)
  line L644 (33.475, 45.475) -> (33.475, 59.525) projected
  line L645 (7.475, 16.975) -> (7.475, 31.025) projected
  line L646 (-39.775, 11.925) -> (-25.725, 11.925) projected
  point P0 (0, 0)
  dimension "d0" = 0.5
  dimension "d1" = 0.5
  dimension "d2" = 0.5
  dimension "d3" = 0.5
  dimension "d4" = 0.25
  dimension "d5" = 0.25
  dimension "d6" = 0.25
  dimension "d7" = 0.25
  dimension "d8" = 0.25
  dimension "d9" = 2
  dimension "d10" = 12.4
  constraints: 78 end point, 20 point on line, 17 perpendicular, 15 collinear, 7 parallel, 2 horizontal, 1 vertical
  measures "d0" distance between parallel lines of L451 L364
  measures "d1" distance between parallel lines of L450 L365
  measures "d2" distance between parallel lines of L449 L366
  measures "d3" distance between parallel lines of L367 L448
  measures "d4" distance between parallel lines of L432 L447
  measures "d5" distance between parallel lines of L446 L431
  measures "d6" distance between parallel lines of L445 L430
  measures "d7" distance between parallel lines of L444 L429
  measures "d8" distance between parallel lines of L443 L428
  measures "d9" distance between parallel lines of L639 L24
  measures "d10" distance between parallel lines of L637 L639
ref_plane "Work Plane1" through (0, 0, 0.5) normal (0, 0, 1) x (1, 0, 0)
extrude "Extrusion2" add sketch "Sketch1" along normal blind 0.5